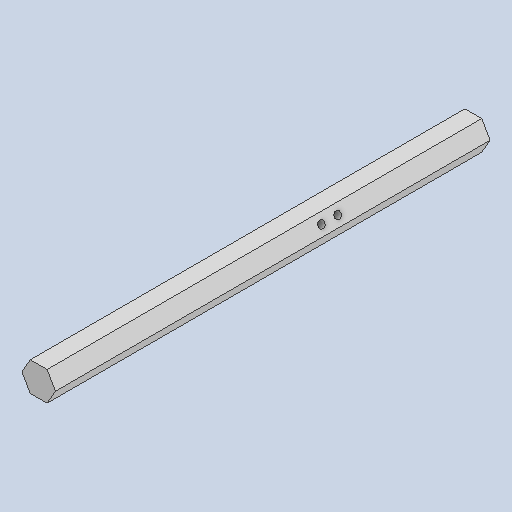
# Autodesk Inventor part: eje3_n
Saved by Autodesk Inventor 2022 (Build 260153000, 153)
## iProperties
Created: 2022-03-11
Part Number: eje3_n
Material: Generic
Document SubType Name: Modeling
Designer: katha
Density: 1 g/cm^3
Appearance: Default
Author: katha
Autodesk Inventor part; units mm, degrees
ref_plane "YZ Plane" through (0, 0, 0) normal (1, 0, 0) x (0, 1, 0)
ref_plane "XZ Plane" through (0, 0, 0) normal (0, 1, 0) x (-1, 0, 0)
ref_plane "XY Plane" through (0, 0, 0) normal (0, 0, 1) x (1, 0, 0)
sketch "Sketch1" plane through (0, 0, 0) normal (0, 0, 1) x (1, 0, 0)
  circle A0 centre (0, 0) radius 7.5 projected
  line L0 (-1.7809, 3.0847) -> (1.7809, 3.0847) projected
  line L1 (0, 0) -> (3.1, 0) construction
  line L2 (0, 0) -> (1.55, 2.6847) construction
  line L3 (0, 0) -> (-1.55, 2.6847) construction
  line L4 (0, 0) -> (-3.1, 0) construction
  line L5 (0, 0) -> (-1.55, -2.6847) construction
  line L6 (0, 0) -> (1.55, -2.6847) construction
  line L7 (-1.55, 2.6847) -> (1.55, 2.6847)
  line L8 (1.55, 2.6847) -> (3.1, 0)
  line L9 (3.1, 0) -> (1.55, -2.6847)
  line L10 (1.55, -2.6847) -> (-1.55, -2.6847)
  line L11 (-1.55, -2.6847) -> (-3.1, 0)
  line L12 (-3.1, 0) -> (-1.55, 2.6847)
  point P0 (0, 0)
  dimension "d0" = 3.1
  dimension "d3" = 360
  constraints: 24 end point, 4 parallel, 2 coincident, 1 horizontal, 17 other
  measures "d0" distance of L1.start L1.end
extrude "Extrusion1" add sketch "Sketch1" against normal blind 80 contours L7 L8 L9 L10 L11 L12
sketch "Sketch2" plane through (3.1, 0, 0) normal (0.866, 0.5, 0) x (0, 0, -1)
  line L0 (0, 3.1) -> (80, 3.1) projected
  line L1 (0, 0) -> (80, 0) projected
  circle A0 centre (49.7, 1.55) radius 0.65
  line L2 (0, 0) -> (0, 3.1) projected
  circle A1 centre (49.7, 7.5397) radius 0.65 projected
  circle A2 centre (52.7, 1.55) radius 0.65
  point P0 (0, 1.55)
  point P1 (0, 1.55)
  dimension "d7" = 1.3
  dimension "d8" = 49.7
  dimension "d9" = 3
  constraints: 2 centre point, 2 horizontal alignment, 1 equal radius, 1 midpoint
  measures "d7" diameter of A0
  measures "d8" distance of point (0, 1.55) A0.centre
  measures "d9" distance of A2.centre A0.centre
extrude "Extrusion3" cut sketch "Sketch2" against normal blind 80 contours A0 | A2
body "Solid1"
